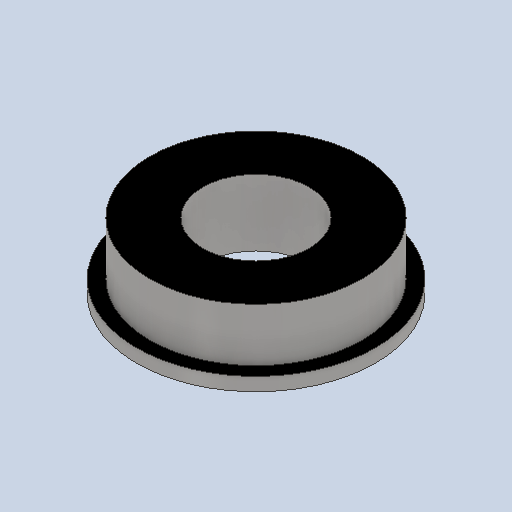
# Autodesk Inventor part: FlangeBearing
Saved by Autodesk Inventor 2022.2 (Build 262287000, 287)
## iProperties
Created: 2022-07-29
Part Number: FlangeBearing
Material: Steel, High Strength, Low Alloy
Document SubType Name: Modeling
Designer: ABL
Density: 7.85 g/cm^3
Appearance: Steel - Polished
Author: ABL
Autodesk Inventor part; units mm, degrees
ref_plane "YZ Plane" through (0, 0, 0) normal (1, 0, 0) x (0, 1, 0)
ref_plane "XZ Plane" through (0, 0, 0) normal (0, 1, 0) x (-1, 0, 0)
ref_plane "XY Plane" through (0, 0, 0) normal (0, 0, 1) x (1, 0, 0)
sketch "Sketch1" plane through (0, 0, 0) normal (0, 0, 1) x (1, 0, 0)
  line L0 (0, 0) -> (0, 5) construction
  line L1 (0, 0) -> (4, 0) construction
  line L2 (4, 0) -> (9, 0)
  line L3 (9, 0) -> (9, 1)
  line L4 (9, 1) -> (8, 1)
  line L5 (8, 1) -> (8, 5)
  line L6 (8, 5) -> (4, 5)
  line L7 (4, 5) -> (4, 0)
  dimension "d2" = 5
  dimension "d5" = 1
  dimension "d7" = 4
  dimension "d9" = 18
  dimension "d10" = 8
  dimension "d11" = 16
  constraints: 16 end point, 5 perpendicular, 1 horizontal, 1 point on line, 1 vertical
  measures "d2" distance of L0.start L0.end
  measures "d5" distance of L2.end L3.end
  measures "d7" distance of L4.end L5.end
  measures "d9" diameter of L3 L0
  measures "d10" diameter of L7 L0
  measures "d11" diameter of L5 L0
revolve "body" add sketch "Sketch1" angle 360 about axis through (0, 0, 0) along (0, 1, 0)
equation "\"d2\" = flangeBearing_height"
equation "\"d5\" = flangeBearing_flangeHeight"
equation "\"d7\" = flangeBearing_height - flangeBearing_flangeHeight"
equation "\"d9\" = flangeBearing_flangeDiameter"
equation "\"d10\" = flangeBearing_innerDiameter"
equation "\"d11\" = flangeBearing_outerDiameter"
equation "\"gap\" = 0.1"
equation "\"airgap\" = 0.4"
equation "\"wallgap\" = 2"
equation "\"driveMagnet_height\" = 5"
equation "\"halbachMagnet_height\" = 3"
equation "\"sensorMagnet_diameter\" = 5"
equation "\"sensorMagnet_height\" = 2.66667"
equation "\"motorRadius\" = 2 * gap + driveMagnet_centerSpacingRadius + driveMagnet_length + 2 * wallgap"
equation "\"shaftDiameter\" = 8"
equation "\"flangeBearing_outerDiameter\" = 16"
equation "\"flangeBearing_innerDiameter\" = shaftDiameter"
equation "\"flangeBearing_height\" = 5"
equation "\"flangeBearing_flangeHeight\" = 1"
equation "\"flangeBearing_flangeDiameter\" = 18"
equation "\"magnetTrapNut_height\" = 1.2"
equation "\"magnetTrapNut_sideToSide\" = 4"
equation "\"magnetTrapBolt_headHeight\" = 2"
equation "\"magnetTrapBolt_headDiameter\" = 3.98"
equation "\"magnetTrapBolt_diameter\" = 2"
equation "\"statorThickness\" = coilThickness + 2 * wallgap"
equation "\"rotor_mountingLipHeight\" = 0.5 * statorThickness"
equation "\"magnetTrapHexNut_sideToSide\" = 4"
equation "\"magnetTrapSquareNut_sideLength\" = 4"
equation "\"magnetTrapSquareNut_height\" = 1.2"
equation "\"magnetTrapHexNut_height\" = 1.2"
equation "\"rotorRadius\" = 2 * gap + driveMagnet_centerSpacingRadius + driveMagnet_length + wallgap"
equation "\"rotorBandSquareNut_sideLength\" = 4"
equation "\"rotorBandHexNut_height\" = 1.2"
equation "\"rotorBandHexNut_sideToSide\" = 4"
equation "\"rotorBandSquareNut_height\" = 1.2"
equation "\"rotorBandBolt_headHeight\" = 2"
equation "\"rotorBandBolt_headDiameter\" = 3.98"
equation "\"rotorBandBolt_diameter\" = 2"
equation "\"rotorBandThickness\" = wallgap + rotorBandBolt_headHeight + gap"
equation "\"flangeCoupling_collarOuterDiameter\" = 16"
equation "\"flangeCoupling_flangeHoleEdgeToEdge\" = 2.05"
equation "\"flangeCoupling_innerDiameter\" = shaftDiameter"
equation "\"flangeCoupling_flangeHoleDiameter\" = 3.9"
equation "\"flangeCoupling_flangeHeight\" = 3.1"
equation "\"flangeCoupling_flangeDiameter\" = 32"
equation "\"flangeCoupling_height\" = flangeCoupling_collarHeight + flangeCoupling_flangeHeight"
equation "\"flangeCoupling_mountHoleDiameter\" = 3.9"
equation "\"flangeCoupling_mountHoleEdgeToEdge\" = 2.05"
equation "\"statorRadius\" = driveMagnet_length + driveMagnet_centerSpacingRadius + 2 * gap"
equation "\"coilThickness\" = 12"
equation "\"statorMountBolt_diameter\" = 4"
equation "\"statorMountBolt_headDiameter\" = 7"
equation "\"statorMountBolt_headHeight\" = 4"
equation "\"statorMountBolt_shaftLength\" = coilThickness + flangeCoupling_flangeHeight + wallgap"
equation "\"statorMountHexNut_height\" = 4"
equation "\"statorMountHexNut_sideToSide\" = 8"
equation "\"sensorMagnet_ringRadius\" = 0.5 * driveMagnet_centerSpacingRadius + 2 * wallgap"
equation "\"coil_percentCoverage\" = 0.6"
equation "\"statorSpokeDegrees\" = 4deg"
equation "\"coil_bulge\" = 3"
equation "\"statorCoilBolt_shaftLength\" = coilThickness"
equation "\"statorCoilHexNut_height\" = 1.2"
equation "\"statorCoilBolt_headHeight\" = 2"
equation "\"statorCoilBolt_diameter\" = 2"
equation "\"statorCoilBolt_headDiameter\" = 3.98"
equation "\"statorCoilHexNut_sideToSide\" = 4"
equation "\"magnetWire_outerDiameter\" = 0.8128"
equation "\"printingLayerHeight\" = 0.2"
equation "\"circuitBoard_height\" = 1.6"
equation "\"hallEffectSensor_width\" = 1.6"
equation "\"hallEffectSensor_length\" = 3"
equation "\"hallEffectSensor_height\" = 1.1"
equation "\"hallEffectSensor_pinLength\" = 0.6"
equation "\"circuitboardMountHexNut_height\" = 1.2"
equation "\"circuitboardMountHexNut_sideToSide\" = 4"
equation "\"circuitboardMountBolt_headHeight\" = 2"
equation "\"circuitboardMountBolt_shaftLength\" = coilThickness"
equation "\"circuitboardMountBolt_diameter\" = 2"
equation "\"circuitboardMountBolt_headDiameter\" = 3.98"
equation "\"statorShellBolt_headDiameter\" = 5.68"
equation "\"statorShellHexNut_height\" = 2.3"
equation "\"statorShellBolt_shaftLength\" = statorThickness - statorShellBolt_countersinkDepth"
equation "\"statorShellBolt_headHeight\" = 3"
equation "\"statorShellHexNut_sideToSide\" = 5.3"
equation "\"statorShellBolt_diameter\" = 3"
equation "\"driveMagnet_centerSpacingRadius\" = 38.96113"
equation "\"driveMagnet_length\" = 60"
equation "\"flangeCoupling_collarHeight\" = 10"
equation "\"statorShellBolt_countersinkDepth\" = 3.4"
